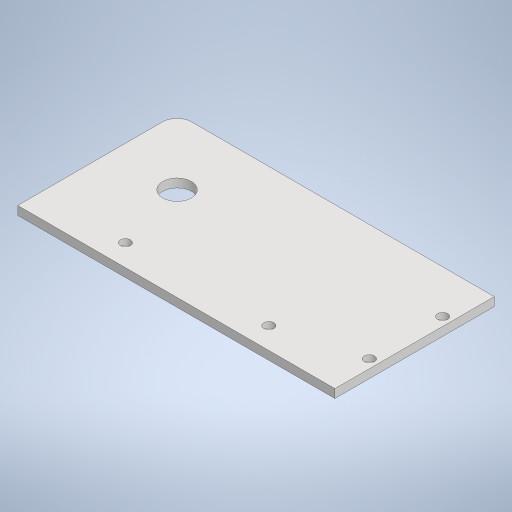
# Autodesk Inventor part: 底板_C
Saved by Autodesk Inventor 2023 (Build 270158000, 158)
## iProperties
Created: 2024-06-09
Part Number: 底板_C
Material: 常规
Document SubType Name: Modeling
Designer: Nitrene.P.L
Density: 1 g/cm^3
Appearance: 默认
Author: Nitrene.P.L
Autodesk Inventor part; units mm, degrees
ref_plane "YZ Plane" through (0, 0, 0) normal (1, 0, 0) x (0, 1, 0)
ref_plane "XZ Plane" through (0, 0, 0) normal (0, 1, 0) x (-1, 0, 0)
ref_plane "XY Plane" through (0, 0, 0) normal (0, 0, 1) x (1, 0, 0)
sketch "草图1" plane through (0, 0, 0) normal (0, 1, 0) x (-1, 0, 0)
  line L0 (110.5, 55.5) -> (-110.5, 55.5)
  line L1 (-110.5, 55.5) -> (-110.5, -55.5)
  line L2 (-110.5, -55.5) -> (110.5, -55.5)
  line L3 (110.5, -55.5) -> (110.5, 55.5)
  line L4 (0, 7.5575) -> (0, -11)
  line L5 (8.5019, 0) -> (-7, 0)
  point P0 (0, 0)
  point P1 (0, 0)
  point P2 (0, 0)
  dimension "d0" = 221
  dimension "d1" = 111
  constraints: 12 end point, 2 horizontal, 2 parallel, 2 vertical, 1 perpendicular, 2 other
  measures "d0" distance of L2.end L1.end
  measures "d1" distance of L1.end L0.end
extrude "拉伸1" add sketch "草图1" along normal blind 6
fillet "圆角1" radius 10.1 1 edges at (-110.5, 3, -55.5)
sketch "草图2" plane through (0, 6, 0) normal (0, 1, 0) x (1, 0, 0)
  circle A0 centre (-64.5, 9.5) radius 10.05
  line L0 (110.5, 55.5) -> (-100.4, 55.5) projected
  line L1 (-110.5, 45.4) -> (-110.5, -55.5) projected
  point P0 (0, 0)
  dimension "d5" = 20.1
  dimension "d6" = 46
  dimension "d7" = 46
  constraints: 1 centre point
  measures "d5" diameter of A0
  measures "d6" distance from line of L0 A0.centre
  measures "d7" distance from line of L1 A0.centre
extrude "拉伸2" cut sketch "草图2" against normal blind 6
sketch "草图3" plane through (0, 6, 0) normal (0, 1, 0) x (1, 0, 0)
  circle A0 centre (-104.5, 25.5) radius 2.1
  circle A1 centre (-104.5, -25.5) radius 2.1
  line L0 (-110.5, -55.5) -> (-110.5, 55.5)
  line L1 (110.5, -55.5) -> (-110.5, -55.5)
  line L2 (-110.5, 55.5) -> (100.4, 55.5)
  circle A2 centre (104.5, -25.5) radius 2.1
  circle A3 centre (104.5, 25.5) radius 2.1
  line L3 (110.5, -55.5) -> (110.5, 55.5) projected
  point P0 (0, 0)
  point P1 (0, 0)
  dimension "d10" = 4.2
  dimension "d11" = 4.2
  dimension "d12" = 6
  dimension "d13" = 6
  dimension "d14" = 30
  dimension "d15" = 30
  dimension "d16" = 4.2
  dimension "d17" = 4.2
  dimension "d18" = 30
  dimension "d19" = 6
  dimension "d20" = 30
  dimension "d21" = 6
  constraints: 6 end point, 4 centre point
  measures "d10" diameter of A0
  measures "d11" diameter of A1
  measures "d12" distance from line of L0 A0.centre
  measures "d13" distance from line of L0 A1.centre
  measures "d14" distance from line of L1 A1.centre
  measures "d15" distance from line of L2 A0.centre
  measures "d16" diameter of A2
  measures "d17" diameter of A3
  measures "d18" distance from line of L1 A2.centre
  measures "d19" distance from line of L3 A2.centre
  measures "d20" distance from line of L2 A3.centre
  measures "d21" distance from line of L3 A3.centre
extrude "拉伸3" cut sketch "草图3" against normal blind 10 contours A2 | A3
sketch "草图4" plane through (0, 6, 0) normal (0, 1, 0) x (1, 0, 0)
  circle A0 centre (104.5, -25.5) radius 2.1 projected
  circle A1 centre (104.5, -25.5) radius 3.6
  circle A2 centre (104.5, 25.5) radius 2.1 projected
  circle A3 centre (104.5, 25.5) radius 3.6
  point P0 (0, 0)
  dimension "d24" = 7.2
  dimension "d25" = 7.2
  constraints: 2 centre point, 2 coincident
  measures "d24" diameter of A1
  measures "d25" diameter of A3
extrude "拉伸4" cut sketch "草图4" against normal blind 4 contours A0 | A1 | A2 | A3
sketch "草图5" plane through (0, 6, 0) normal (0, 1, 0) x (1, 0, 0)
  circle A0 centre (49.5, -40.5) radius 2.1
  circle A1 centre (-50.5, -40.5) radius 2.1
  line L0 (-110.5, -55.5) -> (110.5, -55.5) projected
  line L1 (-110.5, 45.4) -> (-110.5, -55.5) projected
  point P0 (0, 0)
  dimension "d28" = 4.2
  dimension "d29" = 4.2
  dimension "d30" = 15
  dimension "d31" = 15
  dimension "d32" = 60
  dimension "d33" = 100
  constraints: 2 centre point
  measures "d28" diameter of A0
  measures "d29" diameter of A1
  measures "d30" distance from line of L0 A0.centre
  measures "d31" distance from line of L0 A1.centre
  measures "d32" distance from line of L1 A1.centre
  measures "d33" distance of A0.centre A1.centre
extrude "拉伸5" cut sketch "草图5" against normal blind 6
sketch "草图6" plane through (0, 6, 0) normal (0, 1, 0) x (1, 0, 0)
  circle A0 centre (49.5, -40.5) radius 2.1 projected
  circle A1 centre (49.5, -40.5) radius 3.6
  circle A2 centre (-50.5, -40.5) radius 2.1 projected
  circle A3 centre (-50.5, -40.5) radius 3.6
  point P0 (0, 0)
  dimension "d36" = 7.2
  dimension "d37" = 7.2
  constraints: 2 centre point, 2 coincident
  measures "d36" diameter of A1
  measures "d37" diameter of A3
extrude "拉伸6" cut sketch "草图6" against normal blind 4 contours A0 | A1 | A2 | A3
